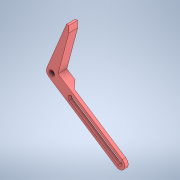
# Autodesk Inventor part: Sliding linkage
Saved by Autodesk Inventor 2020 (Build 240168000, 168)
## iProperties
Created: 2021-06-04
Part Number: Sliding linkage
Material: Generic
Document SubType Name: Modeling
Designer: ugwue
Density: 1 g/cm^3
Appearance: Default
Author: ugwue
Autodesk Inventor part; units mm, degrees
ref_plane "YZ Plane" through (0, 0, 0) normal (1, 0, 0) x (0, 1, 0)
ref_plane "XZ Plane" through (0, 0, 0) normal (0, 1, 0) x (-1, 0, 0)
ref_plane "XY Plane" through (0, 0, 0) normal (0, 0, 1) x (1, 0, 0)
sketch "Sketch2" plane through (0, 0, 0) normal (0, 0, 1) x (1, 0, 0)
  line L0 (-27, 0) -> (18, 0) construction
  circle A0 centre (-42.3909, -42.2862) radius 2.5
  line L1 (-1.368, -72.0925) -> (-26.478, -55.6764)
  arc A1 (-23.742, -51.4914) -> (-26.478, -55.6764) centre (-25.11, -53.5839) ccw
  line L2 (-23.742, -51.4914) -> (1.368, -67.9075)
  arc A2 (-47.0093, -40.3702) -> (-45.1269, -46.4712) centre (-42.3909, -42.2862) ccw
  line L3 (-27, 0) -> (-27, 3)
  line L4 (-27, 3) -> (-27, -3)
  line L5 (-29.0168, 3) -> (-27, 3)
  line L6 (-27, 3) -> (-27, -3)
  line L7 (-29.0168, 3) -> (-47.0093, -40.3702)
  line L8 (-27, -3) -> (-36.781, -39.9801)
  line L9 (-45.1269, -46.4712) -> (-2.736, -74.185)
  line L10 (-36.781, -39.9801) -> (2.736, -65.815)
  line L11 (-2.736, -74.185) -> (15.2131, -85.9196)
  line L12 (2.736, -65.815) -> (21.5936, -78.1435)
  line L13 (15.2131, -85.9196) -> (16.1216, -86.5135)
  arc A3 (16.1216, -86.5135) -> (21.5936, -78.1435) centre (18.8576, -82.3285) ccw
  line L14 (1.368, -67.9075) -> (20.2256, -80.236)
  line L15 (17.4896, -84.421) -> (-1.368, -72.0925)
  arc A4 (17.4896, -84.421) -> (20.2256, -80.236) centre (18.8576, -82.3285) ccw
  point P0 (0, 0)
  constraints: 32 end point, 8 point on circle, 5 centre point, 4 tangent, 3 parallel, 2 coincident, 1 horizontal, 1 point on line, 1 vertical
extrude "Extrusion2" add sketch "Sketch2" along normal blind 8
sketch "Sketch3" plane through (-36.781, -39.9801, 8) normal (0.5472037, 0.8369994, 0) x (0.8369994, -0.5472037, 0)
  line L0 (74.7426, 8) -> (74.7426, 0) projected
  line L1 (8.9084, 8) -> (74.7426, 8)
  line L2 (74.7426, 8) -> (74.7426, 3)
  line L3 (74.7426, 3) -> (13.9084, 3)
  line L4 (8.9084, 8) -> (13.9084, 3)
  line L5 (8.9084, 8) -> (15.9795, 8) construction
  point P0 (74.7426, 8)
  dimension "d30" = 5
  dimension "d31" = 45
  constraints: 10 end point, 2 horizontal, 1 equal length, 1 parallel, 1 perpendicular, 1 point on line
  measures "d30" distance of L1.end L2.end
  measures "d31" angle of L4 L5
extrude "Extrusion3" cut sketch "Sketch3" against normal blind 10
body "Solid2"
